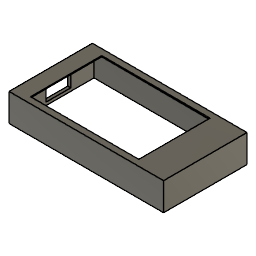
first_test_print_Ben (Autodesk Fusion 360 design; units mm, degrees)
Autodesk Fusion 360 part; units mm, degrees
sketch "Sketch1" plane through (0, 0, 0) normal (0, 0, 1) x (1, 0, 0)
  line L0 (0, 0) -> (127, 0)
  line L1 (127, 0) -> (127, 68.58)
  line L2 (127, 68.58) -> (0, 68.58)
  line L3 (0, 68.58) -> (0, 0)
  line L4 (0, 0) -> (0, 34.29)
  line L5 (0, 34.29) -> (12.7, 34.29)
  line L6 (101.6, 0) -> (101.6, 63.5)
  line L7 (101.6, 63.5) -> (12.7, 63.5)
  line L8 (12.7, 63.5) -> (12.7, 0)
  line L9 (101.6, 5.08) -> (12.7, 5.08)
  dimension "d1" = 127
  dimension "d2" = 68.58
  dimension "d3" = 34.29
  dimension "d4" = 12.7
  dimension "d6" = 63.5
  constraint horizontal L0
  constraint vertical L1
  constraint horizontal L2
  constraint vertical L3
  constraint coincident L0.start L3.end
  constraint perpendicular L0 L4
  constraint perpendicular L3 L5
  constraint coincident L0 L6.start
  constraint perpendicular L0 L6
  constraint perpendicular L3 L7
  constraint coincident L0 L8.end
  constraint perpendicular L0 L8
  constraint coincident L6 L9.start
  constraint coincident L8 L9.end
  constraint perpendicular L8 L9
  measures "d1" distance of L0.start L0.end
  measures "d2" distance of L0.start L2.end
  measures "d3" distance of L0.start L4.end
  measures "d4" distance of L4.end L5.end
  measures "d6" distance of L6.start L6.end
extrude "Extrude1" add sketch "Sketch1" against normal blind 22.86 contours L0 L3 L4 L5 L8 | L0 L6 L8 L9 | L0 L1 L2 L3 L5 L6 L7 L8
sketch "Sketch2" plane through (0, 0, 0) normal (-1, 0, 0) x (0, -1, 0)
  line L0 (0, 0) -> (-68.58, 0)
  line L1 (-68.58, 0) -> (-68.58, -22.86)
  line L2 (-68.58, -22.86) -> (0, -22.86)
  line L3 (0, -22.86) -> (0, 0)
  line L4 (-68.58, -22.86) -> (-68.58, -20.32)
  line L5 (-27.94, -20.32) -> (-27.94, -6.35)
  line L6 (-27.94, -6.35) -> (-48.26, -6.35)
  line L7 (-48.26, -6.35) -> (-48.26, -20.32)
  line L8 (-48.26, -20.32) -> (-27.94, -20.32)
  dimension "d12" = 13.97
  constraint coincident L1.end L2.start
  constraint perpendicular L2 L4
  constraint perpendicular L5 L6
  constraint perpendicular L5 L8
  measures "d12" distance of L5.start L5.end
extrude "Extrude2" cut sketch "Sketch2" against normal blind 5.08 contours L5 L6 L7 L8
sketch "Sketch3" plane through (101.6, 0, 0) normal (-1, 0, 0) x (0, -1, 0)
  line L0 (-5.08, 0) -> (-63.5, 0)
  line L1 (-63.5, 0) -> (-63.5, -22.86)
  line L2 (-63.5, -22.86) -> (-5.08, -22.86)
  line L3 (-5.08, -22.86) -> (-5.08, 0)
  line L4 (-63.5, -22.86) -> (-63.5, -1.27)
  line L5 (-63.5, -1.27) -> (-5.08, -1.27)
  line L6 (-5.08, -22.86) -> (-5.08, -1.27)
  line L7 (-63.5, -22.86) -> (-5.08, -22.86)
  constraint coincident L1.end L2.start
  constraint coincident L1 L4.end
  constraint coincident L3 L5.end
  constraint perpendicular L3 L5
  constraint coincident L2.end L3.start
extrude "Extrude3" cut sketch "Sketch3" against normal blind 22.86 contours L1 L2 L3 L4 L5 L6 L7
sketch "Sketch4" plane through (12.7, 0, 0) normal (1, 0, 0) x (0, 1, 0)
  line L0 (63.5, 0) -> (5.08, 0)
  line L1 (5.08, 0) -> (5.08, -22.86)
  line L2 (5.08, -22.86) -> (63.5, -22.86)
  line L3 (63.5, -22.86) -> (63.5, 0)
  line L4 (5.08, -22.86) -> (5.08, -0.762)
  line L5 (5.08, -0.762) -> (63.5, -0.762)
  line L6 (63.5, -22.86) -> (63.5, -0.762)
  line L7 (63.5, -22.86) -> (5.08, -22.86)
  constraint coincident L1.end L2.start
  constraint coincident L1 L4.end
  constraint coincident L3 L5.end
  constraint perpendicular L3 L5
  constraint coincident L2.end L3.start
extrude "Extrude4" cut sketch "Sketch4" against normal blind 10.16 contours L1 L2 L3 L4 L5 L6 L7
sketch "Sketch5" plane through (0, 63.5, 0) normal (0, -1, 0) x (1, 0, 0)
  line L0 (101.6, 0) -> (12.7, 0)
  line L1 (12.7, 0) -> (12.7, -0.762)
  line L2 (12.7, -0.762) -> (2.54, -0.762)
  line L3 (2.54, -0.762) -> (2.54, -22.86)
  line L4 (2.54, -22.86) -> (124.46, -22.86)
  line L5 (124.46, -22.86) -> (124.46, -1.27)
  line L6 (124.46, -1.27) -> (101.6, -1.27)
  line L7 (101.6, -1.27) -> (101.6, 0)
  line L8 (2.54, -0.762) -> (124.46, -1.27)
  line L9 (124.46, -22.86) -> (2.54, -22.86)
  line L10 (2.54, -0.762) -> (2.54, -21.3653)
  constraint coincident L2.end L3.start
  constraint coincident L5.end L6.start
  constraint coincident L4.end L5.start
  constraint coincident L3.end L4.start
  constraint coincident L3 L10.end
extrude "Extrude5" cut sketch "Sketch5" against normal blind 3.81 contours L3 L4 L5 L6 L7 L8 L9 L10
sketch "Sketch6" plane through (0, 5.08, 0) normal (0, 1, 0) x (-1, 0, 0)
  line L0 (-12.7, 0) -> (-101.6, 0)
  line L1 (-101.6, 0) -> (-101.6, -1.27)
  line L2 (-101.6, -1.27) -> (-124.46, -1.27)
  line L3 (-124.46, -1.27) -> (-124.46, -22.86)
  line L4 (-124.46, -22.86) -> (-2.54, -22.86)
  line L5 (-2.54, -22.86) -> (-2.54, -0.762)
  line L6 (-2.54, -0.762) -> (-12.7, -0.762)
  line L7 (-12.7, -0.762) -> (-12.7, 0)
  line L8 (-124.46, -1.27) -> (-2.54, -0.762)
  line L9 (-2.54, -22.86) -> (-124.46, -22.86)
  line L10 (-124.46, -1.27) -> (-124.46, -22.86)
  constraint coincident L2.end L3.start
  constraint coincident L5.end L6.start
  constraint coincident L4.end L5.start
  constraint coincident L3.end L4.start
extrude "Extrude6" cut sketch "Sketch6" against normal blind 3.81 contours L1 L2 L3 L4 L5 L8 L9 L10
